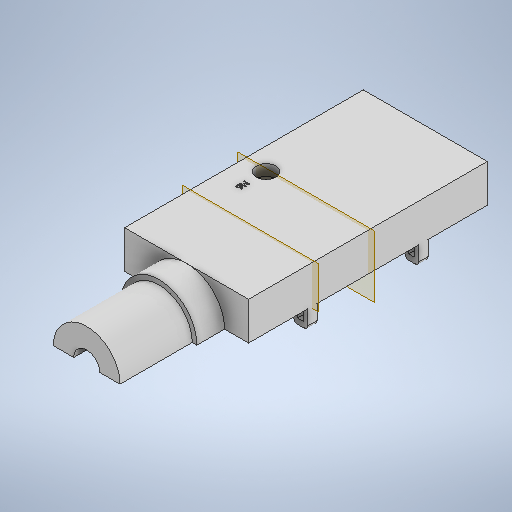
# Autodesk Inventor part: Pen_Housing_Top_V2
Saved by Autodesk Inventor 2025 (Build 290162000, 162)
## iProperties
Created: 2024-05-28
Part Number: Pen_Housing_Top_V2
Material: Generic
Document SubType Name: Modeling
Designer: mumin
Density: 1 g/cm^3
Appearance: Default
Author: mumin
Autodesk Inventor part; units mm, degrees
ref_plane "YZ Plane" through (0, 0, 0) normal (1, 0, 0) x (0, 1, 0)
ref_plane "XZ Plane" through (0, 0, 0) normal (0, 1, 0) x (-1, 0, 0)
sketch "Sketch1" plane through (0, 0, 0) normal (1, 0, 0) x (0, 1, 0)
  line L0 (0, -64.5) -> (20.5, -64.5)
  line L1 (20.5, -64.5) -> (20.5, 64.5)
  line L2 (20.5, 64.5) -> (0, 64.5)
  line L3 (0, 64.5) -> (0, -64.5)
  line L4 (0, -64.5) -> (20.5, 64.5) construction
  line L5 (20.5, -64.5) -> (0, 64.5) construction
  point P0 (0, 0)
  point P1 (10.25, 0)
  dimension "d0" = 129
  dimension "d1" = 20.5
  constraints: 12 end point, 3 midpoint, 2 parallel, 1 horizontal, 1 perpendicular
  measures "d0" distance of L0.end L1.end
  measures "d1" distance of L1.end L2.end
extrude "Extrusion1" add sketch "Sketch1" along normal mid plane 67
sketch "Sketch2" plane through (-33.5, 0, 64.5) normal (0, 0, 1) x (1, 0, 0)
  line L0 (0, 0) -> (67, 0) projected
  arc A0 (54, 0) -> (13, 0) centre (33.5, 0) ccw
  point P0 (13, 0)
  dimension "d4" = 20.5
  constraints: 2 point on circle, 1 centre point, 1 coincident, 1 point on line
  measures "d4" radius of A0
extrude "Extrusion2" add sketch "Sketch2" along normal blind 15
sketch "Sketch3" plane through (-33.5, 0, 79.5) normal (0, 0, 1) x (1, 0, 0)
  line L0 (0, 0) -> (67, 0) projected
  arc A0 (51.5, 0) -> (15.5, 0) centre (33.5, 0) ccw
  line L1 (33.5, 0) -> (15.5, 0) construction
  line L2 (33.5, 0) -> (51.5, 0) construction
  point P0 (15.5, 0)
  dimension "d7" = 18
  dimension "d8" = 180
  constraints: 4 end point, 2 point on circle, 1 centre point, 1 coincident, 1 point on line
  measures "d7" radius of A0
  measures "d8" angle of L1 L2
extrude "Extrusion3" add sketch "Sketch3" along normal blind 39
sketch "Sketch5" plane through (33.5, 20.5, -64.5) normal (0, 0, -1) x (-1, 0, 0)
  arc A0 (40.5, -20.5) -> (26.5, -20.5) centre (33.5, -20.5) ccw
  line L0 (33.5, -20.5) -> (26.5, -20.5) construction
  line L1 (33.5, -20.5) -> (40.5, -20.5) construction
  line L2 (67, -20.5) -> (0, -20.5) projected
  point P0 (26.5, -20.5)
  dimension "d16" = 7
  dimension "d17" = 180
  constraints: 4 end point, 2 point on circle, 1 centre point, 1 coincident, 1 point on line
  measures "d16" radius of A0
  measures "d17" angle of L0 L1
extrude "Extrusion5" cut sketch "Sketch5" against normal through all
ref_plane "Work Plane1" through (0, 0, 30) normal (0, 0, 1) x (1, 0, 0)
sketch "Sketch6" plane through (0, 0, 30) normal (0, 0, 1) x (1, 0, 0)
  line L0 (33.5, 0) -> (33.5, -8)
  line L1 (31, -7.0278) -> (31, -2)
  line L2 (31.5, -10) -> (28, -10)
  line L3 (26, -8) -> (26, -5)
  arc A0 (27.9998, -7.0278) -> (26, -5) centre (26, -7) ccw
  line L4 (31, -7.0278) -> (27.9998, -7.0278)
  arc A1 (31, -2) -> (29, 0) centre (29, -2) ccw
  arc A2 (31.5, -10) -> (33.5, -8) centre (31.5, -8) ccw
  arc A3 (26, -8) -> (28, -10) centre (28, -8) ccw
  line L5 (7, 0) -> (33.5, 0) projected
  line L6 (33.5, 0) -> (33.5, 20.5) projected
  point P0 (0, 0)
  point P1 (33.5, -10)
  point P2 (31, -0.0278)
  point P3 (26, -10)
  point P4 (29, 0)
  dimension "d21" = 10
  dimension "d22" = 2.5
  dimension "d23" = 7
  dimension "d24" = 7.5
  dimension "d25" = 5
  dimension "d26" = 2
  dimension "d27" = 2
  dimension "d28" = 2
  constraints: 10 end point, 8 point on circle, 6 point on line, 5 tangent, 4 centre point, 1 equal radius
  measures "d21" distance of L0.start point (33.5, -10)
  measures "d22" distance between parallel lines of L0 L1
  measures "d23" distance of L4.start point (31, -0.028)
  measures "d24" distance of point (33.5, -10) point (26, -10)
  measures "d25" distance of point (26, -10) L3.end
  measures "d26" distance of L3.end A0.centre
  measures "d27" radius of A1
  measures "d28" radius of A2
extrude "Extrusion6" add sketch "Sketch6" along normal mid plane 5
mirror "Mirror1" about plane through (0, 0, 0) normal (0, 0, 1) of "Extrusion6"
sketch "Sketch7" plane through (-33.5, 20.5, -64.5) normal (0, 1, 0) x (1, 0, 0)
  line L0 (80.4, -64.5) -> (-13.4, -64.5) projected
  line L1 (0, -129) -> (0, 0) projected
  point P0 (33.5, -64.5)
  point P1 (12, -64.5)
  dimension "d38" = 12
  constraints: 1 point on line
  measures "d38" distance from line of L1 point (12, -64.5)
hole "Hole1" at (-21.5, 20.5, 0) direction (0, -1, 0) diameter 6.2 end through all counterbore diameter 10.5 counterbore depth 6
sketch "Sketch8" plane through (-33.5, 20.5, -64.5) normal (0, 1, 0) x (1, 0, 0)
  line L0 (13.4766, -74.3991) -> (13.4766, -79.9171) construction
  line L1 (13.4766, -79.9171) -> (5.3533, -79.9171) construction
  line L2 (5.3533, -79.9171) -> (5.3533, -74.3991) construction
  line L3 (5.3533, -74.3991) -> (13.4766, -74.3991) construction
  line L4 (10.3718, -77.3212) -> (10.3718, -76.9161)
  line L5 (10.3718, -76.9161) -> (12.9974, -76.9161)
  line L6 (12.9974, -76.9161) -> (11.2116, -76.1207)
  line L7 (11.2116, -76.1207) -> (11.2116, -75.8737)
  line L8 (11.2116, -75.8737) -> (12.9974, -75.0858)
  line L9 (12.9974, -75.0858) -> (10.3718, -75.0858)
  line L10 (10.3718, -75.0858) -> (10.3718, -74.7079)
  line L11 (10.3718, -74.7079) -> (13.4198, -74.7079)
  line L12 (13.4198, -74.7079) -> (13.4198, -75.2612)
  line L13 (13.4198, -75.2612) -> (11.7229, -76.0219)
  line L14 (11.7229, -76.0219) -> (13.4198, -76.758)
  line L15 (13.4198, -76.758) -> (13.4198, -77.3212)
  line L16 (13.4198, -77.3212) -> (10.3718, -77.3212)
  spline S0 degree 2 poles (11.3598, -79.7788) (11.1252, -79.7788) (10.7275, -79.6232) (10.5941, -79.4923) knots 0 0 0 1 2 2 2
  spline S1 degree 2 poles (10.5941, -79.4923) (10.4533, -79.3564) (10.3076, -79.0156) (10.3076, -78.8106) knots 0 0 0 1 2 2 2
  spline S2 degree 2 poles (10.3076, -78.8106) (10.3076, -78.6056) (10.4459, -78.2672) (10.5842, -78.1387) knots 0 0 0 1 2 2 2
  spline S3 degree 2 poles (10.5842, -78.1387) (10.7497, -77.9806) (11.3055, -77.8028) (11.7105, -77.8028) knots 0 0 0 1 2 2 2
  spline S4 degree 2 poles (11.7105, -77.8028) (12.1082, -77.8028) (12.748, -77.9658) (12.9851, -78.1363) knots 0 0 0 1 2 2 2
  spline S5 degree 2 poles (12.9851, -78.1363) (13.2173, -78.3017) (13.4766, -78.8254) (13.4766, -79.1687) knots 0 0 0 1 2 2 2
  spline S6 degree 2 poles (13.4766, -79.1687) (13.4766, -79.27) (13.4568, -79.4478) (13.4346, -79.5145) knots 0 0 0 1 2 2 2
  line L17 (13.4346, -79.5145) -> (13.0419, -79.5145)
  line L18 (13.0419, -79.5145) -> (13.0419, -79.4972)
  spline S7 degree 2 poles (13.0419, -79.4972) (13.0715, -79.4404) (13.1234, -79.2329) (13.1234, -79.1144) knots 0 0 0 1 2 2 2
  spline S8 degree 2 poles (13.1234, -79.1144) (13.1234, -78.734) (12.6096, -78.2672) (12.1057, -78.2227) knots 0 0 0 1 2 2 2
  spline S9 degree 2 poles (12.1057, -78.2227) (12.207, -78.3684) (12.3182, -78.6747) (12.3182, -78.8575) knots 0 0 0 1 2 2 2
  spline S10 degree 2 poles (12.3182, -78.8575) (12.3182, -79.0353) (12.2465, -79.3021) (12.1379, -79.4478) knots 0 0 0 1 2 2 2
  spline S11 degree 2 poles (12.1379, -79.4478) (12.0119, -79.6158) (11.6216, -79.7788) (11.3598, -79.7788) knots 0 0 0 1 2 2 2
  spline S12 degree 2 poles (11.3425, -79.3639) (11.5302, -79.3639) (11.7846, -79.2651) (11.8736, -79.1564) knots 0 0 0 1 2 2 2
  spline S13 degree 2 poles (11.8736, -79.1564) (11.9378, -79.0749) (11.9798, -78.8723) (11.9798, -78.7661) knots 0 0 0 1 2 2 2
  spline S14 degree 2 poles (11.9798, -78.7661) (11.9798, -78.6228) (11.8933, -78.3536) (11.8118, -78.2227) knots 0 0 0 1 2 2 2
  spline S15 degree 2 poles (11.8118, -78.2227) (11.7674, -78.2202) (11.6834, -78.2153) (11.6192, -78.2153) knots 0 0 0 1 2 2 2
  spline S16 degree 2 poles (11.6192, -78.2153) (11.303, -78.2153) (10.9152, -78.3388) (10.8139, -78.4327) knots 0 0 0 1 2 2 2
  spline S17 degree 2 poles (10.8139, -78.4327) (10.7176, -78.5191) (10.641, -78.7068) (10.641, -78.813) knots 0 0 0 1 2 2 2
  spline S18 degree 2 poles (10.641, -78.813) (10.641, -79.06) (10.9918, -79.3639) (11.3425, -79.3639) knots 0 0 0 1 2 2 2
  point P0 (33.5, -64.5)
  constraints: 2 other
emboss "Emboss1" sketch "Sketch8" operation cut depth 1 direction (0, -1, 0)
body "Solid1"
